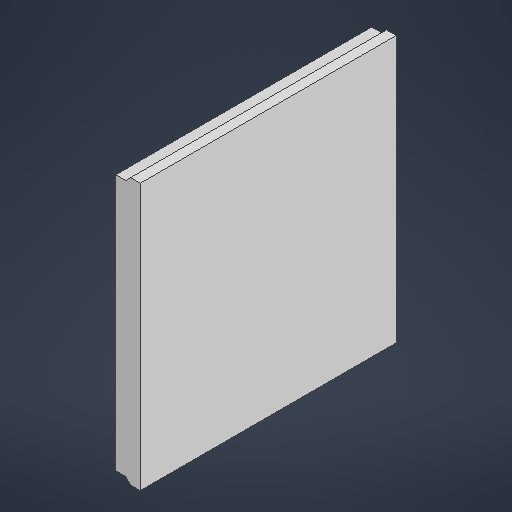
# Autodesk Inventor part: battery holder lid
Saved by Autodesk Inventor 2025.2 (Build 292293000, 293)
## iProperties
Created: 2025-05-21
Part Number: battery holder lid
Material: Generic
Document SubType Name: Modeling
Designer: klawy
Density: 1 g/cm^3
Appearance: Default
Author: klawy
Autodesk Inventor part; units mm, degrees
ref_plane "YZ Plane" through (0, 0, 0) normal (1, 0, 0) x (0, 1, 0)
ref_plane "XZ Plane" through (0, 0, 0) normal (0, 1, 0) x (-1, 0, 0)
ref_plane "XY Plane" through (0, 0, 0) normal (0, 0, 1) x (1, 0, 0)
sketch "Sketch1" plane through (0, 0, 0) normal (0, 1, 0) x (-1, 0, 0)
  line L0 (-20, -25) -> (20, -25) construction
  line L1 (20, -25) -> (20, 25) construction
  line L2 (20, 25) -> (-20, 25) construction
  line L3 (-20, 25) -> (-20, -25) construction
  line L4 (-20, -25) -> (20, 25) construction
  line L5 (20, -25) -> (-20, 25) construction
  line L6 (25, 30) -> (25, -30)
  line L7 (25, -30) -> (-25, -30)
  line L8 (-25, -30) -> (-25, 30)
  line L9 (-25, 30) -> (25, 30)
  point P0 (0, 0)
  dimension "d0" = 50
  dimension "d1" = 40
  dimension "d2" = 5
  constraints: 20 end point, 4 parallel, 2 midpoint, 2 perpendicular, 1 horizontal, 3 other
  measures "d0" distance of L0.end L1.end
  measures "d1" distance of L1.end L2.end
  measures "d2" distance between parallel lines of L1 L6
sketch "Sketch2" plane through (0, 0, 0) normal (0, 1, 0) x (-1, 0, 0)
  line L0 (-20, -25) -> (20, -25) construction
  line L1 (20, -25) -> (20, 25) construction
  line L2 (20, 25) -> (-20, 25) construction
  line L3 (-20, 25) -> (-20, -25) construction
  line L4 (-20, -25) -> (20, 25) construction
  line L5 (20, -25) -> (-20, 25) construction
  line L6 (25, 30) -> (25, -30) projected
  line L7 (25, -30) -> (-25, -30) projected
  line L8 (-25, -30) -> (-25, 30) projected
  line L9 (-25, 30) -> (25, 30) projected
  point P0 (0, 0)
  point P1 (0, 0)
extrude "Extrusion1" add sketch "Sketch1" against normal blind 3
hole "Hole1" at (20, 0, -25) at (-20, 0, 25) at (-20, 0, -25) at (20, 0, 25) direction (0, -1, 0) diameter 3.4 end through all clearance for "Socket Head Cap Screw ISO 4762" size "M3" standard "ISO"
fillet "Fillet1" radius 2 4 edges at (25, -1.5, 30) (-25, -1.5, 30) (25, -1.5, -30) (-25, -1.5, -30)
sketch "Sketch3" plane through (0, 0, 0) normal (0, 1, 0) x (1, 0, 0)
  circle A0 centre (4.95, 16.1) radius 7.05
  line L0 (4.95, 37.6221) -> (4.95, -37.6221) construction
  circle A1 centre (4.95, 0) radius 7.05
  circle A2 centre (4.95, -16.1) radius 7.05
  line L1 (15, -26.15) -> (-5.1, -26.15)
  line L2 (-5.1, -26.15) -> (-5.1, 26.15)
  line L3 (-5.1, 26.15) -> (15, 26.15)
  line L4 (15, 26.15) -> (15, -26.15)
  line L5 (15, -26.15) -> (-5.1, 26.15) construction
  line L6 (-5.1, -26.15) -> (15, 26.15) construction
  line L7 (35, 0) -> (-35, 0) projected
  line L8 (25, -28) -> (25, 28) projected
  line L9 (4.95, 23.15) -> (-5.1, 23.15)
  line L10 (4.95, 9.05) -> (-5.1, 9.05)
  line L11 (4.95, 7.05) -> (-5.1, 7.05)
  line L12 (4.95, -7.05) -> (-5.3479, -7.05)
  line L13 (4.95, -9.05) -> (-5.1, -9.05)
  line L14 (4.95, -23.15) -> (-5.1, -23.15)
  point P0 (4.95, 26.15)
  point P1 (-5.1, -7.05)
  dimension "d15" = 14.1
  dimension "d16" = 14.1
  dimension "d17" = 14.1
  dimension "d18" = 16.1
  dimension "d19" = 16.1
  dimension "d20" = 10.05
  dimension "d21" = 10.05
  dimension "d60" = 10
  constraints: 24 end point, 6 perpendicular, 6 point on circle, 6 point on line, 6 tangent, 3 centre point, 3 midpoint, 3 parallel, 1 horizontal, 12 other
  measures "d15" diameter of A0
  measures "d16" diameter of A1
  measures "d17" diameter of A2
  measures "d18" distance of A1.centre A0.centre
  measures "d19" distance of A1.centre A2.centre
  measures "d20" distance of point (4.95, 26.15) A0.centre
  measures "d21" distance from line of L2 A0.centre
  measures "d60" distance between parallel lines of L8 L4
extrude "Extrusion2" add sketch "Sketch3" along normal blind 50.5 contours A0 L9 L2 L3 L4 L7 A1 L11 L10 | L4 L1 L2 L14 A2 L13 L12 A1 L7
sketch "Sketch4" plane through (0, -3, 0) normal (0, -1, 0) x (1, 0, 0)
  line L0 (15, -26.15) -> (-5.1, -26.15) projected
  line L1 (-5.1, -26.15) -> (-5.1, -23.15) projected
  line L2 (-5.1, 26.15) -> (15, 26.15) projected
  line L3 (15, 26.15) -> (15, -26.15) projected
  arc A0 (4.95, 9.05) -> (4.95, 23.15) centre (4.95, 16.1) ccw projected
  arc A1 (4.95, -7.05) -> (4.95, 7.05) centre (4.95, 0) ccw projected
  arc A2 (4.95, -23.15) -> (4.95, -9.05) centre (4.95, -16.1) ccw projected
  circle A3 centre (4.95, -16.1) radius 1
  circle A4 centre (4.95, 16.1) radius 1
  line L4 (-5.1, -23.15) -> (4.95, -23.15) projected
  line L5 (4.95, -9.05) -> (-5.1, -9.05) projected
  line L6 (-5.1, -9.05) -> (-5.1, -7.05) projected
  line L7 (-5.1, -7.05) -> (4.95, -7.05) projected
  line L8 (4.95, 7.05) -> (-5.1, 7.05) projected
  line L9 (-5.1, 7.05) -> (-5.1, 9.05) projected
  line L10 (-5.1, 9.05) -> (4.95, 9.05) projected
  line L11 (4.95, 23.15) -> (-5.1, 23.15) projected
  line L12 (-5.1, 23.15) -> (-5.1, 26.15) projected
  point P0 (0, 0)
  dimension "d24" = 2
  dimension "d25" = 2
  constraints: 2 centre point, 2 coincident
  measures "d24" diameter of A3
  measures "d25" diameter of A4
sketch "Sketch5" plane through (4.95, 0, -16.1) normal (0, 1, 0) x (0, 0, -1)
  line L0 (10.05, -10.05) -> (10.05, 10.05) projected
  line L1 (10.05, 10.05) -> (7.05, 10.05) projected
  line L2 (-42.25, 10.05) -> (-42.25, -10.05) projected
  line L3 (-42.25, -10.05) -> (10.05, -10.05) projected
  arc A0 (-39.25, 0) -> (-25.15, 0) centre (-32.2, 0) ccw projected
  arc A1 (-23.15, 0) -> (-9.05, 0) centre (-16.1, 0) ccw projected
  arc A2 (-7.05, 0) -> (7.05, 0) centre (0, 0) ccw projected
  circle A3 centre (0, 0) radius 2.5
  line L4 (7.05, 10.05) -> (7.05, 0) projected
  line L5 (-7.05, 0) -> (-7.05, 10.05) projected
  line L6 (-7.05, 10.05) -> (-9.05, 10.05) projected
  line L7 (-9.05, 10.05) -> (-9.05, 0) projected
  line L8 (-23.15, 0) -> (-23.15, 10.05) projected
  line L9 (-23.15, 10.05) -> (-25.15, 10.05) projected
  line L10 (-25.15, 10.05) -> (-25.15, 0) projected
  line L11 (-39.25, 0) -> (-39.25, 10.05) projected
  line L12 (-39.25, 10.05) -> (-42.25, 10.05) projected
  point P0 (-16.1, 4.95)
  dimension "d26" = 5
  constraints: 1 centre point, 1 coincident
  measures "d26" diameter of A3
extrude "Extrusion3" cut sketch "Sketch5" against normal blind 1 contours A3
extrude "Extrusion4" cut sketch "Sketch4" against normal blind 2 contours A3
sketch "Sketch7" plane through (0, 50.5, 0) normal (0, 1, 0) x (1, 0, 0)
  line L0 (15, 26.15) -> (-5.1, 26.15) projected
  line L1 (-5.1, 26.15) -> (-5.1, 23.15) projected
  line L2 (-5.1, -26.15) -> (15, -26.15) projected
  line L3 (15, -26.15) -> (15, 26.15) projected
  arc A0 (4.95, -23.15) -> (4.95, -9.05) centre (4.95, -16.1) ccw construction
  arc A1 (4.95, -7.05) -> (4.95, 7.05) centre (4.95, 0) ccw construction
  arc A2 (4.95, 9.05) -> (4.95, 23.15) centre (4.95, 16.1) ccw construction
  line L4 (-5.1, 23.15) -> (4.95, 23.15) projected
  line L5 (4.95, 9.05) -> (-5.1, 9.05) projected
  line L6 (-5.1, 9.05) -> (-5.1, 7.05) projected
  line L7 (-5.1, 7.05) -> (4.95, 7.05) projected
  line L8 (4.95, -7.05) -> (-5.1, -7.05) projected
  line L9 (-5.1, -7.05) -> (-5.1, -9.05) projected
  line L10 (-5.1, -9.05) -> (4.95, -9.05) projected
  line L11 (4.95, -23.15) -> (-5.1, -23.15) projected
  line L12 (-5.1, -23.15) -> (-5.1, -26.15) projected
  line L13 (-5.1, 26.15) -> (15, 26.15)
  line L14 (15, 26.15) -> (15, -26.15)
  line L15 (15, -26.15) -> (-5.1, -26.15)
  line L16 (-5.1, -26.15) -> (-5.1, 26.15)
  point P0 (0, 0)
  point P1 (-5.1, -23.15)
  constraints: 8 end point, 2 parallel, 1 horizontal, 1 perpendicular
extrude "Extrusion5" add sketch "Sketch7" along normal blind 8
sketch "Sketch14" plane through (0, 50.5, 0) normal (0, -1, 0) x (1, 0, 0)
  line L0 (-5.1, -23.15) -> (4.95, -23.15) projected
  arc A0 (4.95, -23.15) -> (4.95, -9.05) centre (4.95, -16.1) ccw projected
  line L1 (4.95, -9.05) -> (-5.1, -9.05) projected
  line L2 (-5.1, -23.15) -> (-5.1, -9.05) projected
  line L3 (4.95, 7.05) -> (-5.1, 7.05) projected
  line L4 (-5.1, -7.05) -> (-5.1, 7.05) projected
  line L5 (-5.1, -7.05) -> (4.95, -7.05) projected
  arc A1 (4.95, -7.05) -> (4.95, 7.05) centre (4.95, 0) ccw projected
  line L6 (4.95, 23.15) -> (-5.1, 23.15) projected
  line L7 (-5.1, 9.05) -> (-5.1, 23.15) projected
  line L8 (-5.1, 9.05) -> (4.95, 9.05) projected
  arc A2 (4.95, 9.05) -> (4.95, 23.15) centre (4.95, 16.1) ccw projected
  circle A3 centre (4.95, -16.1) radius 2.5
  circle A4 centre (4.95, 0) radius 2.5
  circle A5 centre (4.95, 16.1) radius 2.5
  point P0 (0, 0)
  dimension "d66" = 5
  dimension "d67" = 5
  dimension "d68" = 5
  constraints: 3 centre point, 3 coincident
  measures "d66" diameter of A3
  measures "d67" diameter of A4
  measures "d68" diameter of A5
extrude "Extrusion10" cut sketch "Sketch14" against normal blind 1 contours A3 | A4 | A5
sketch "Sketch15" plane through (4.95, 51.5, -16.1) normal (0, -1, 0) x (1, 0, 0)
  circle A0 centre (0, 0) radius 2.5 construction
  circle A1 centre (0, 16.1) radius 2.5 construction
  line L0 (-2.5, 0) -> (-2.5, 16.1)
  line L1 (2.5, 16.1) -> (2.5, 0)
  line L2 (0, 0) -> (0, 16.1) construction
  line L3 (2.5, 0) -> (-2.5, 0)
  line L4 (2.5, 16.1) -> (-2.5, 16.1)
  point P0 (-4.95, 16.1)
  constraints: 10 end point, 4 point on circle, 3 parallel, 2 tangent, 2 vertical, 1 horizontal
extrude "Extrusion11" cut sketch "Sketch15" against normal blind 2
chamfer "Chamfer1" distance 2 angle 45 2 edges at (4.95, 51.5, 0) (4.95, 51.5, -16.1)
sketch "Sketch16" plane through (0, 0, 0) normal (0, 1, 0) x (1, 0, 0)
  circle A0 centre (4.95, 16.1) radius 2.5 projected
  line L0 (-5.1, 26.15) -> (15, 26.15) projected
  line L1 (15, 26.15) -> (15, -26.15) projected
  line L2 (15, -26.15) -> (-5.1, -26.15) projected
  line L3 (-5.1, -26.15) -> (-5.1, -23.15) projected
  line L4 (-5.1, -23.15) -> (4.95, -23.15) projected
  arc A1 (4.95, -23.15) -> (4.95, -9.05) centre (4.95, -16.1) ccw projected
  line L5 (4.95, -9.05) -> (-5.1, -9.05) projected
  line L6 (-5.1, -9.05) -> (-5.1, -7.05) projected
  line L7 (-5.1, -7.05) -> (4.95, -7.05) projected
  arc A2 (4.95, -7.05) -> (4.95, 7.05) centre (4.95, 0) ccw projected
  line L8 (4.95, 7.05) -> (-5.1, 7.05) projected
  line L9 (-5.1, 7.05) -> (-5.1, 9.05) projected
  line L10 (-5.1, 9.05) -> (4.95, 9.05) projected
  arc A3 (4.95, 9.05) -> (4.95, 23.15) centre (4.95, 16.1) ccw projected
  line L11 (4.95, 23.15) -> (-5.1, 23.15) projected
  line L12 (-5.1, 23.15) -> (-5.1, 26.15) projected
  circle A4 centre (20, -25) radius 1.7 projected
  circle A5 centre (-20, 25) radius 1.7 projected
  circle A6 centre (-20, -25) radius 1.7 projected
  circle A7 centre (20, 25) radius 1.7 projected
  arc A8 (-23, 30) -> (-25, 28) centre (-23, 28) ccw projected
  line L13 (-25, 28) -> (-25, -28) projected
  arc A9 (-25, -28) -> (-23, -30) centre (-23, -28) ccw projected
  line L14 (-23, -30) -> (23, -30) projected
  arc A10 (23, -30) -> (25, -28) centre (23, -28) ccw projected
  line L15 (25, -28) -> (25, 28) projected
  arc A11 (25, 28) -> (23, 30) centre (23, 28) ccw projected
  line L16 (23, 30) -> (-23, 30) projected
  circle A12 centre (4.95, 0) radius 2.5
  circle A13 centre (4.95, -16.1) radius 2.5
  line L17 (5.95, -2.2913) -> (5.95, -13.8087)
  line L18 (3.95, -13.8087) -> (3.95, -2.2913)
  line L19 (4.95, 0) -> (4.95, -16.1) construction
  point P0 (0, 0)
  dimension "d76" = 5
  dimension "d77" = 5
  dimension "d78" = 2
  dimension "d79" = 1
  constraints: 6 end point, 4 point on circle, 2 centre point, 2 coincident, 2 vertical, 1 parallel
  measures "d76" diameter of A12
  measures "d77" diameter of A13
  measures "d78" distance between parallel lines of L18 L17
  measures "d79" distance between parallel lines of L19 L18
extrude "Extrusion12" cut sketch "Sketch16" against normal blind 1 contours L17 A13 L18 L5 A1 | A1 L5 L18 L7 A2 L17 | A2 L7 L18 A12 L17 | A13 | A12
sketch "Sketch17" plane through (4.95, 51.5, 16.1) normal (0, -1, 0) x (1, 0, 0)
  circle A0 centre (0, -32.2) radius 1 projected
  arc A1 (-29.95, -44.1) -> (-27.95, -46.1) centre (-27.95, -44.1) ccw projected
  line L0 (-27.95, -46.1) -> (18.05, -46.1) projected
  arc A2 (18.05, -46.1) -> (20.05, -44.1) centre (18.05, -44.1) ccw projected
  line L1 (20.05, -44.1) -> (20.05, 11.9) projected
  arc A3 (20.05, 11.9) -> (18.05, 13.9) centre (18.05, 11.9) ccw projected
  line L2 (18.05, 13.9) -> (-27.95, 13.9) projected
  arc A4 (-27.95, 13.9) -> (-29.95, 11.9) centre (-27.95, 11.9) ccw projected
  line L3 (-29.95, 11.9) -> (-29.95, -44.1) projected
  circle A5 centre (15.05, 8.9) radius 1.7 projected
  circle A6 centre (-24.95, -41.1) radius 1.7 projected
  circle A7 centre (-24.95, 8.9) radius 1.7 projected
  circle A8 centre (15.05, -41.1) radius 1.7 projected
  circle A9 centre (0, -16.1) radius 2.5 projected
  circle A10 centre (0, 0) radius 2.5 construction
  line L4 (0, 0) -> (7.05, -7.05) construction
  line L5 (-10.05, -7.05) -> (-10.05, 7.05) projected
  circle A11 centre (7.05, -7.05) radius 1.5
  line L6 (0, -7.05) -> (-1, -7.05) projected
  line L7 (-10.05, -7.05) -> (0, -7.05) projected
  line L8 (-1, -7.05) -> (-10.05, -7.05) projected
  arc A12 (1, -6.9787) -> (0, 7.05) centre (0, 0) ccw projected
  arc A13 (0, -7.05) -> (0, 7.05) centre (0, 0) ccw projected
  arc A14 (0, -7.05) -> (1, -6.9787) centre (0, 0) ccw projected
  line L9 (1, -13.8087) -> (1, -9.1213) projected
  arc A15 (0, -23.15) -> (1, -9.1213) centre (0, -16.1) ccw projected
  line L10 (0, -23.15) -> (-10.05, -23.15) projected
  line L11 (-10.05, -23.15) -> (-10.05, -25.15) projected
  line L12 (-10.05, -25.15) -> (0, -25.15) projected
  arc A16 (0, -39.25) -> (0, -25.15) centre (0, -32.2) ccw projected
  line L13 (0, -39.25) -> (-10.05, -39.25) projected
  line L14 (-10.05, -39.25) -> (-10.05, -42.25) projected
  line L15 (-10.05, -42.25) -> (10.05, -42.25) projected
  line L16 (10.05, -42.25) -> (10.05, 10.05) projected
  line L17 (10.05, 10.05) -> (-10.05, 10.05) projected
  line L18 (-10.05, 10.05) -> (-10.05, 7.05) projected
  line L19 (-10.05, 7.05) -> (0, 7.05) projected
  arc A17 (1, -6.9787) -> (0, 7.05) centre (0, 0) ccw projected
  line L20 (1, -6.9787) -> (1, -2.2913) projected
  arc A18 (1, -2.2913) -> (-1, -2.2913) centre (0, 0) ccw projected
  line L21 (-1, -2.2913) -> (-1, -7.05) projected
  line L22 (-1, -7.05) -> (-10.05, -7.05) projected
  line L23 (-10.05, -7.05) -> (-10.05, -9.05) projected
  line L24 (-10.05, -9.05) -> (-1, -9.05) projected
  line L25 (-1, -9.05) -> (-1, -13.8087) projected
  arc A19 (-1, -13.8087) -> (1, -13.8087) centre (0, -16.1) ccw projected
  circle A20 centre (0, -32.2) radius 2.5 projected
  circle A21 centre (15.05, 8.9) radius 1.7 projected
  circle A22 centre (-24.95, -41.1) radius 1.7 projected
  circle A23 centre (-24.95, 8.9) radius 1.7 projected
  circle A24 centre (15.05, -41.1) radius 1.7 projected
  arc A25 (-29.95, -44.1) -> (-27.95, -46.1) centre (-27.95, -44.1) ccw projected
  line L26 (-29.95, -44.1) -> (-29.95, 11.9) projected
  arc A26 (-27.95, 13.9) -> (-29.95, 11.9) centre (-27.95, 11.9) ccw projected
  line L27 (-27.95, 13.9) -> (18.05, 13.9) projected
  arc A27 (20.05, 11.9) -> (18.05, 13.9) centre (18.05, 11.9) ccw projected
  line L28 (20.05, 11.9) -> (20.05, -44.1) projected
  arc A28 (18.05, -46.1) -> (20.05, -44.1) centre (18.05, -44.1) ccw projected
  line L29 (18.05, -46.1) -> (-27.95, -46.1) projected
  point P0 (-4.95, -16.1)
  dimension "d83" = 3
  dimension "d84" = 45
  dimension "d85" = 3
  constraints: 2 end point, 1 centre point
  measures "d83" diameter of A11
  measures "d84" angle of L20 L4
  measures "d85" distance from line of L16 L4.end
extrude "Extrusion13" cut sketch "Sketch17" along normal through all contours A11
sketch "Sketch18" plane through (4.95, 51.5, 16.1) normal (0, -1, 0) x (1, 0, 0)
  circle A0 centre (7.05, -7.05) radius 1.5 projected
  circle A1 centre (7.05, -7.05) radius 1.5 projected
  circle A2 centre (0, 0) radius 2.5 projected
  circle A3 centre (0, 0) radius 2.5 projected
  line L0 (7.05, -7.05) -> (0, 0) construction
  line L1 (8.1107, -5.9893) -> (2.4749, -0.3536)
  circle A4 centre (0, 0) radius 2.5 projected
  line L2 (0.3536, -2.4749) -> (5.9893, -8.1107)
  line L3 (0.3536, -2.4749) -> (2.4749, -0.3536)
  line L4 (8.1107, -5.9893) -> (5.9893, -8.1107)
  point P0 (-4.95, -16.1)
  point P1 (5.2928, -3.1714)
  point P2 (5.9893, -8.1107)
  dimension "d89" = 3
  constraints: 10 end point, 4 point on circle, 3 parallel, 1 midpoint, 2 other
  measures "d89" distance from line of L2 point (5.293, -3.171)
extrude "Extrusion14" cut sketch "Sketch18" against normal blind 2 contours L4 A0 | A0 L2 A2 L1 | A2 L3 picked at (6.5012, -6.2587) picked at (1.7238, -1.2336)
chamfer "Chamfer2" distance 2 angle 45 1 edges at (6.3642, 51.5, 14.6858)
chamfer "Chamfer3" distance 1.4 angle 45 1 edges at (12, 51.5, 9.05)
sketch "Sketch19" plane through (0, 0, 0) normal (0, 1, 0) x (1, 0, 0)
  line L0 (5.95, -2.2913) -> (5.95, -13.8087) projected
  arc A0 (5.95, -2.2913) -> (3.95, -2.2913) centre (4.95, 0) ccw projected
  line L1 (3.95, -13.8087) -> (3.95, -2.2913) projected
  arc A1 (3.95, -13.8087) -> (5.95, -13.8087) centre (4.95, -16.1) ccw projected
  circle A2 centre (4.95, -16.1) radius 7.05
  line L2 (-5.1, -9.05) -> (-5.1, -7.05) projected
  line L3 (-5.1, -23.15) -> (4.95, -23.15) projected
  line L4 (-5.1, -9.05) -> (-5.1, -23.15)
  point P0 (0, 0)
  dimension "d98" = 14.1
  constraints: 2 end point, 1 coincident, 1 vertical, 1 vertical alignment, 1 other
sketch "Sketch20" plane through (-5.1, 50.5, -23.15) normal (-1, 0, 0) x (0, 0, 1)
  line L0 (49.3, -50.5) -> (46.3, -50.5) projected
  line L1 (49.3, -50.5) -> (49.3, 8) projected
  line L2 (-3, 8) -> (49.3, 8) projected
  line L3 (-3, -50.5) -> (-3, 8) projected
  line L4 (0, -50.5) -> (-3, -50.5) projected
  line L5 (0, -50.5) -> (0, 0) projected
  line L6 (0, 0) -> (14.1, 0) projected
  line L7 (14.1, -50.5) -> (14.1, 0) projected
  line L8 (16.1, -50.5) -> (14.1, -50.5) projected
  line L9 (16.1, -50.5) -> (16.1, 0) projected
  line L10 (16.1, 0) -> (30.2, 0) projected
  line L11 (30.2, -50.5) -> (30.2, 0) projected
  line L12 (32.2, -50.5) -> (30.2, -50.5) projected
  line L13 (32.2, -50.5) -> (32.2, 0) projected
  line L14 (32.2, 0) -> (46.3, 0) projected
  line L15 (46.3, -50.5) -> (46.3, 0) projected
  point P0 (23.15, -50.5)
extrude "Extrusion15" add sketch "Sketch20" along normal blind 2
sketch "Sketch21" plane through (0, 0, 0) normal (0, 1, 0) x (1, 0, 0)
  line L0 (-7.1, -23.15) -> (4.95, -23.15) projected
  line L1 (-7.1, -23.15) -> (-7.1, 23.15)
  line L2 (-2.1, -23.15) -> (-2.1, 23.15)
  circle A0 centre (4.95, -16.1) radius 7.05 projected
  line L3 (4.95, 23.15) -> (-7.1, 23.15) projected
  point P0 (0, 0)
  constraints: 4 end point, 2 point on line, 2 vertical, 1 vertical alignment
extrude "Extrusion16" add sketch "Sketch21" along normal blind 58.5 contours L1 L3 L2 L0
sketch "Sketch22" plane through (15, 0, 26.15) normal (0, 0, 1) x (1, 0, 0)
  line L0 (-22.1, 0) -> (-22.1, 58.5) projected
  line L1 (-22.1, 29.25) -> (0.0273, 29.25) construction
  line L2 (-22.1, 0) -> (-22.1, 3)
  line L3 (-22.1, 3) -> (-20.1, 3) construction
  line L4 (-20.1, 3) -> (-19.1, 2) construction
  line L5 (-19.1, 2) -> (-17.1, 2) construction
  line L6 (-17.1, 2) -> (-17.1, 0)
  line L7 (-11.05, 0) -> (-17.1, 0) projected
  line L8 (-38, 0) -> (8, 0) projected
  line L9 (-22.1, 58.5) -> (-22.1, 0)
  line L10 (-22.1, 58.5) -> (-22.1, 55.5)
  line L11 (-22.1, 55.5) -> (-20.1, 55.5) construction
  line L12 (-20.1, 55.5) -> (-19.1, 56.5) construction
  line L13 (-19.1, 56.5) -> (-17.1, 56.5) construction
  line L14 (-17.1, 56.5) -> (-17.1, 58.5)
  line L15 (-11.05, 58.5) -> (-17.1, 58.5)
  line L16 (-17.1, 2) -> (-17.1, 56.5)
  line L17 (-61.1197, 77.7276) -> (44.0103, 77.7276)
  line L18 (44.0103, 77.7276) -> (44.0103, -41.1524)
  line L19 (44.0103, -41.1524) -> (-61.1197, -41.1524)
  line L20 (-61.1197, -41.1524) -> (-61.1197, 77.7276)
  line L21 (-17.1, 56.45) -> (-19.0793, 56.45)
  line L22 (-19.0793, 56.45) -> (-20.0793, 55.45)
  line L23 (-20.0793, 55.45) -> (-22.1, 55.45)
  line L24 (-17.1, 2.05) -> (-19.0793, 2.05)
  line L25 (-19.0793, 2.05) -> (-20.0793, 3.05)
  line L26 (-20.0793, 3.05) -> (-22.1, 3.05)
  point P0 (-15, 0)
  point P1 (-15, 58.5)
  dimension "d104" = 3
  dimension "d105" = 2
  dimension "d106" = 2
  dimension "d107" = 45
  dimension "d108" = 5
  dimension "d111" = 0.05
  dimension "d112" = 0.05
  dimension "d113" = 0.05
  dimension "d114" = 0.05
  dimension "d115" = 0.05
  dimension "d116" = 0.05
  constraints: 48 end point, 10 symmetric about line, 8 point on line, 5 parallel, 5 perpendicular, 4 horizontal, 1 collinear, 1 midpoint
  measures "d104" distance of L0.start L2.end
  measures "d105" distance of L2.end L3.end
  measures "d106" distance of L4.end L5.end
  measures "d107" angle of L8 L4
  measures "d108" distance of L0.start L6.end
  measures "d111" distance between parallel lines of L13 L21
  measures "d112" distance between parallel lines of L12 L22
  measures "d113" distance between parallel lines of L11 L23
  measures "d114" distance between parallel lines of L5 L24
  measures "d115" distance between parallel lines of L4 L25
  measures "d116" distance between parallel lines of L3 L26
extrude "Extrusion17" cut sketch "Sketch22" along normal through all both and the other way through all contours L0 L26 L25 L24 L16 L6 L8 | L17 L18 L19 L20
equation "\"d16\" = d15"
equation "\"d17\" = d15"
equation "\"d19\" = d18"
equation "\"d21\" = d20"
body "Solid1"
